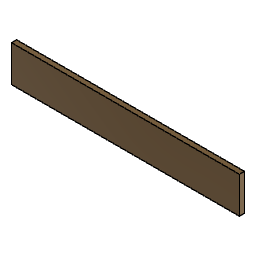
control_panel_front (Autodesk Fusion 360 design; units mm, degrees)
Autodesk Fusion 360 part; units mm, degrees
sketch "Control Panel Front" plane through (0, 0, 0) normal (0, 1, 0) x (1, 0, 0)
  line L0 (0, 0) -> (270, 0)
  line L1 (270, 0) -> (270, -43)
  line L2 (270, -43) -> (0, -43)
  line L3 (0, -43) -> (0, 0)
  dimension "d6" = 270
  dimension "d7" = 43
  constraint horizontal L0
  constraint vertical L1
  constraint horizontal L2
  constraint vertical L3
  constraint coincident L0.start L3.end
  measures "d6" distance of L0.start L0.end
  measures "d7" distance of L0.end L1.end
extrude "Extrude1" add sketch "Control Panel Front" along normal blind 6
equation "MDFThickness = 6 mm" comment "Thickness of the MDF board"
equation "d2 = MDFThickness"
equation "d7 = sidePanelControlPanelHeight - 2 * sidePanelClearance - 2 * MDFThickness"
equation "sidePanelClearance = 10 mm" comment "Clearance between side panel edge and main body edge"
equation "sidePanelControlPanelHeight = 75 mm" comment "The height of the control panel on the side panel"
named bodies: "Control Panel Front"
